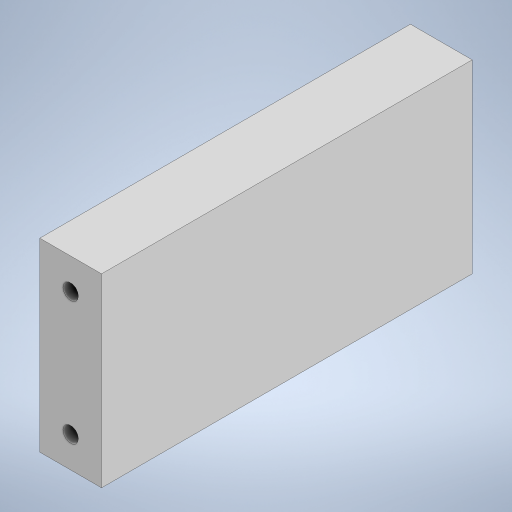
# Autodesk Inventor part: ベースパーツ_実験装置取り付け部分
Saved by Autodesk Inventor 2024.3 (Build 283343000, 343)
## iProperties
Created: 2024-10-09
Part Number: ベースパーツ_実験装置取り付け部分
Material: 一般
Document SubType Name: Modeling
Designer: hikou
Density: 1 g/cm^3
Appearance: 既定
Author: hikou
Autodesk Inventor part; units mm, degrees
ref_plane "YZ Plane" through (0, 0, 0) normal (1, 0, 0) x (0, 1, 0)
ref_plane "XZ Plane" through (0, 0, 0) normal (0, 1, 0) x (-1, 0, 0)
ref_plane "XY Plane" through (0, 0, 0) normal (0, 0, 1) x (1, 0, 0)
sketch "スケッチ1" plane through (0, 0, 0) normal (0, 0, 1) x (1, 0, 0)
  line L0 (-5, -15) -> (5, -15)
  line L1 (5, -15) -> (5, 15)
  line L2 (5, 15) -> (-5, 15)
  line L3 (-5, 15) -> (-5, -15)
  line L4 (-5, -15) -> (5, 15) construction
  line L5 (5, -15) -> (-5, 15) construction
  point P0 (0, 0)
  dimension "d0" = 10
  dimension "d1" = 30
  constraints: 12 end point, 2 midpoint, 2 parallel, 1 horizontal, 1 perpendicular
  measures "d0" distance of L2.end L1.end
  measures "d1" distance of L0.end L1.end
extrude "押し出し1" add sketch "スケッチ1" along normal mid plane 60
sketch "スケッチ2" plane through (0, 0, 30) normal (0, 0, 1) x (1, 0, 0)
  line L0 (5, 15) -> (-5, 15) projected
  line L1 (5, -15) -> (5, 15) projected
  line L2 (-5, -15) -> (5, -15) projected
  point P0 (0, 0)
  point P1 (0, 10)
  point P2 (0, -10)
  dimension "d4" = 5
  dimension "d5" = 5
  dimension "d6" = 5
  dimension "d7" = 5
  measures "d4" distance from line of L0 point (0, 10)
  measures "d5" distance from line of L1 point (0, 10)
  measures "d6" distance from line of L1 point (0, -10)
  measures "d7" distance from line of L2 point (0, -10)
hole "穴1" at (0, 10, 30) at (0, -10, 30) direction (0, 0, -1) diameter 2.5 end through all
equation "\"d5\" = d4"
equation "\"d6\" = d4"
equation "\"d7\" = d4"
